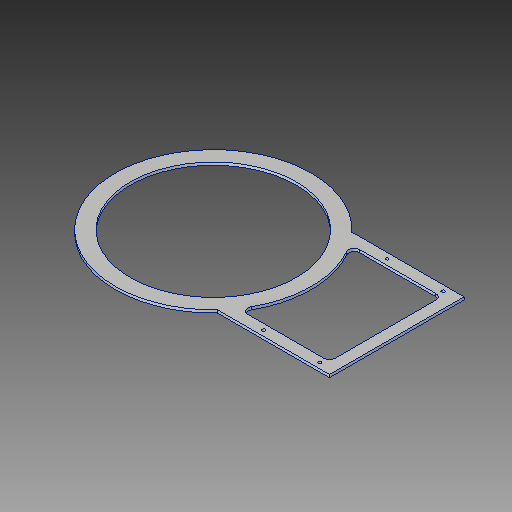
# Autodesk Inventor part: Turret Support 2
Saved by Autodesk Inventor 2019.4 (Build 234330000, 330)
## iProperties
Created: 2020-01-19
Part Number: Turret Support 2
Material: Aluminum 6061
Document SubType Name: Modeling
Designer: Mark
Mass: 528.483 g
Surface Area: 941.759 cm^2
Volume: 195.734 cm^3
Density: 2.7 g/cm^3
Appearance: Aluminum - Flat
Author: Mark
Autodesk Inventor part; units mm, degrees
ref_plane "YZ Plane" through (0, 0, 0) normal (1, 0, 0) x (0, 1, 0)
ref_plane "XZ Plane" through (0, 0, 0) normal (0, 1, 0) x (-1, 0, 0)
ref_plane "XY Plane" through (0, 0, 0) normal (0, 0, 1) x (1, 0, 0)
sketch "Sketch1" plane through (0, 0, 0) normal (0, 1, 0) x (-1, 0, 0)
  circle A0 centre (0, 0) radius 175
  circle A1 centre (0, 0) radius 148
  dimension "d0" = 350
  dimension "d1" = 296
  constraints: 2 centre point, 2 coincident
  measures "d0" diameter of A0
  measures "d1" diameter of A1
extrude "Extrusion1" add sketch "Sketch1" along normal blind 5
sketch "Sketch2" plane through (0, 5, 0) normal (0, 1, 0) x (1, 0, 0)
  circle A0 centre (0, 0) radius 175 projected
  line L0 (-127.3774, -120) -> (127.3774, -120)
  line L1 (127.3774, -120) -> (127.3774, 120)
  line L2 (127.3774, 120) -> (-127.3774, 120)
  line L3 (-127.3774, 120) -> (-127.3774, -120)
  line L4 (-127.3774, -120) -> (127.3774, 120) construction
  line L5 (127.3774, -120) -> (-127.3774, 120) construction
  line L6 (127.3774, -120) -> (327.3774, -120)
  line L7 (327.3774, -120) -> (327.3774, 120)
  line L8 (327.3774, 120) -> (127.3774, 120)
  line L9 (127.3774, 120) -> (127.3774, -120)
  dimension "d4" = 240
  dimension "d5" = 200
  dimension "d6" = 240
  constraints: 20 end point, 4 parallel, 2 horizontal, 2 midpoint, 2 perpendicular, 1 point on circle
  measures "d4" distance of L0.end L1.end
  measures "d5" distance of L8.end L7.end
  measures "d6" distance of L7.end L6.end
extrude "Extrusion2" add sketch "Sketch2" against normal blind 5 contours A0 L1 | A0 L8 L7 L6
sketch "Sketch3" plane through (0, 5, 0) normal (0, 1, 0) x (1, 0, 0)
  circle A0 centre (0, 0) radius 148
  line L0 (327.3774, 120) -> (327.3774, -120) projected
  line L1 (327.3774, 100) -> (167.3774, 100)
  line L2 (167.3774, -100) -> (327.3774, -100)
  line L3 (327.3774, -100) -> (327.3774, 100)
  line L4 (327.3774, 120) -> (127.3774, 120) projected
  line L5 (127.3774, -120) -> (327.3774, -120) projected
  arc A1 (127.3774, 120) -> (127.3774, -120) centre (0, 0) ccw projected
  arc A2 (143.6141, -100) -> (143.6141, 100) centre (0, 0) ccw
  line L6 (167.3774, 100) -> (143.6141, 100)
  line L7 (167.3774, -100) -> (143.6141, -100)
  dimension "d9" = 296
  dimension "d10" = 20
  dimension "d11" = 20
  dimension "d12" = 160
  dimension "d16" = 175
  constraints: 10 end point, 2 centre point, 2 horizontal, 2 point on circle, 1 coincident, 1 collinear, 1 concentric, 1 parallel, 1 point on line
  measures "d9" diameter of A0
  measures "d10" distance between parallel lines of L4 L1
  measures "d11" distance between parallel lines of L5 L2
  measures "d12" distance of L2.start L2.end
  measures "d16" radius of A2
extrude "Extrusion3" cut sketch "Sketch3" against normal blind 5 contours A0 | L0 L2 L7 A2 L6 L1
fillet "Fillet1" radius 10 2 edges at (143.6141, 2.5, -100) (143.6141, 2.5, 100)
sketch "Sketch4" plane through (0, 5, 0) normal (0, 1, 0) x (1, 0, 0)
  line L0 (327.3774, -120) -> (327.3774, -100) projected
  line L1 (327.3774, -100) -> (307.3774, -100)
  line L2 (307.3774, -100) -> (307.3774, 100)
  line L3 (307.3774, 100) -> (327.3774, 100)
  line L4 (327.3774, 100) -> (327.3774, -100)
  point P0 (0, 0)
  dimension "d17" = 20
  dimension "d18" = 200
  constraints: 8 end point, 2 parallel, 1 horizontal, 1 perpendicular
  measures "d17" distance of L2.end L3.end
  measures "d18" distance of L1.end L2.end
extrude "Extrusion4" add sketch "Sketch4" against normal blind 5
fillet "Fillet2" radius 10 2 edges at (307.3774, 2.5, 100) (307.3774, 2.5, -100)
sketch "Sketch5" plane through (0, 5, 0) normal (0, 1, 0) x (1, 0, 0)
  circle A0 centre (300.0004, 110) radius 2.75
  circle A1 centre (200.0004, 110) radius 2.75
  circle A2 centre (300.0004, -110) radius 2.75
  circle A3 centre (200.0004, -110) radius 2.75
  line L0 (127.3774, -120) -> (327.3774, -120) projected
  line L1 (327.3774, 120) -> (127.3774, 120) projected
  line L2 (327.3774, -120) -> (327.3774, 120) projected
  point P0 (0, 0)
  dimension "d22" = 5.5
  dimension "d23" = 5.5
  dimension "d24" = 5.5
  dimension "d25" = 5.5
  dimension "d26" = 100
  dimension "d27" = 10
  dimension "d28" = 10
  dimension "d29" = 10
  dimension "d30" = 10
  dimension "d31" = 100
  dimension "d32" = 27.377
  dimension "d33" = 27.377
  constraints: 4 centre point
  measures "d22" diameter of A0
  measures "d23" diameter of A1
  measures "d24" diameter of A2
  measures "d25" diameter of A3
  measures "d26" distance of A2.centre A3.centre
  measures "d27" distance from line of L0 A2.centre
  measures "d28" distance from line of L0 A3.centre
  measures "d29" distance from line of L1 A0.centre
  measures "d30" distance from line of L1 A1.centre
  measures "d31" distance of A0.centre A1.centre
  measures "d32" distance from line of A0.centre L2
  measures "d33" distance from line of L2 A2.centre
extrude "Extrusion5" cut sketch "Sketch5" against normal blind 10
body "Solid1"
